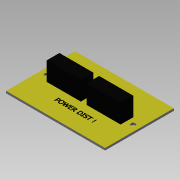
# Autodesk Inventor part: powerdiset
Saved by Autodesk Inventor 2015 SP1 (Build 190203100, 203)
## iProperties
Created: 2015-01-28
Part Number: powerdiset
Material: Generic
Document SubType Name: Modeling
Designer: Rafi Kurnia Putra
Density: 1 g/cm^3
Appearance: Default
Author: Rafi Kurnia Putra
Autodesk Inventor part; units mm, degrees
ref_plane "YZ Plane" through (0, 0, 0) normal (1, 0, 0) x (0, 1, 0)
ref_plane "XZ Plane" through (0, 0, 0) normal (0, 1, 0) x (-1, 0, 0)
ref_plane "XY Plane" through (0, 0, 0) normal (0, 0, 1) x (1, 0, 0)
sketch "Sketch1" plane through (0, 0, 0) normal (0, 1, 0) x (-1, 0, 0)
  line L0 (39.28, 27.305) -> (-39.28, 27.305)
  line L1 (-39.28, 27.305) -> (-39.28, -27.305)
  line L2 (-39.28, -27.305) -> (39.28, -27.305)
  line L3 (39.28, -27.305) -> (39.28, 27.305)
  line L4 (39.28, 27.305) -> (-39.28, -27.305) construction
  line L5 (-39.28, 27.305) -> (39.28, -27.305) construction
  circle A0 centre (-34.28, 0) radius 1.75
  circle A1 centre (34.28, 0) radius 1.75
  line L6 (29.28, -5) -> (2.28, -5)
  line L7 (2.28, -5) -> (2.28, 5)
  line L8 (2.28, 5) -> (29.28, 5)
  line L9 (29.28, 5) -> (29.28, -5)
  line L10 (29.28, -5) -> (2.28, 5) construction
  line L11 (2.28, -5) -> (29.28, 5) construction
  line L12 (-29.28, 5) -> (-2.28, 5)
  line L13 (-2.28, 5) -> (-2.28, -5)
  line L14 (-2.28, -5) -> (-29.28, -5)
  line L15 (-29.28, -5) -> (-29.28, 5)
  line L16 (-29.28, 5) -> (-2.28, -5) construction
  line L17 (-2.28, 5) -> (-29.28, -5) construction
  point P0 (0, 0)
  point P1 (15.78, 0)
  point P2 (-15.78, 0)
  dimension "d0" = 78.56
  dimension "d1" = 54.61
  dimension "d2" = 3.5
  dimension "d3" = 5
  dimension "d4" = 3.5
  dimension "d5" = 5
  dimension "d6" = 27
  dimension "d7" = 10
  dimension "d8" = 5
  dimension "d9" = 27
  dimension "d10" = 10
  dimension "d11" = 5
  dimension "d16" = 68.56
  constraints: 36 end point, 6 midpoint, 6 parallel, 3 horizontal, 3 perpendicular, 2 centre point
  measures "d0" distance of L2.end L1.end
  measures "d1" distance of L1.end L0.end
  measures "d2" diameter of A0
  measures "d3" distance from line of A0.centre L1
  measures "d4" diameter of A1
  measures "d5" distance from line of A1.centre L3
  measures "d6" distance of L7.end L8.end
  measures "d7" distance of L6.end L7.end
  measures "d8" distance from line of L9 A1.centre
  measures "d9" distance of L13.end L14.end
  measures "d10" distance of L12.end L13.end
  measures "d11" distance from line of L15 A0.centre
  measures "d16" distance of A0.centre A1.centre
extrude "Extrusion1" add sketch "Sketch1" along normal blind 1.7
extrude "Extrusion2" add sketch "Sketch1" along normal blind 16.58 contours L6 L7 L8 L9 | L12 L13 L14 L15
sketch "Sketch2" plane through (0, 1.7, 0) normal (0, 1, 0) x (1, 0, 0)
  line L0 (-13.9986, -11.26) -> (17.2433, -11.26) construction
  line L1 (17.2433, -11.26) -> (17.2433, -14.9075) construction
  line L2 (17.2433, -14.9075) -> (-13.9986, -14.9075) construction
  line L3 (-13.9986, -14.9075) -> (-13.9986, -11.26) construction
  point P0 (0, 0)
  constraints: 2 other
body "Solid1"
